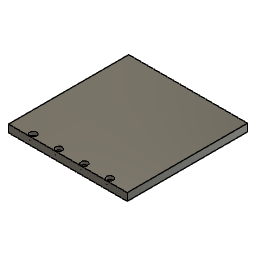
PlaceHeadCover v3 (Autodesk Fusion 360 design; units mm, degrees)
Autodesk Fusion 360 part; units mm, degrees
sketch "Sketch1" plane through (0, 0, 0) normal (0, 1, 0) x (1, 0, 0)
  line L0 (0, 0) -> (79, 0)
  line L1 (79, 0) -> (79, -80)
  line L2 (79, -80) -> (0, -80)
  line L3 (0, -80) -> (0, 0)
  dimension "d1" = 79
  dimension "d2" = 80
  constraint horizontal L0
  constraint vertical L1
  constraint horizontal L2
  constraint vertical L3
  constraint coincident L0.start L3.end
  measures "d1" distance of L0.start L0.end
  measures "d2" distance of L0.start L2.end
extrude "Extrude1" add sketch "Sketch1" along normal blind 5
sketch "Sketch2" plane through (0, 5, 0) normal (0, 1, 0) x (-1, 0, 0)
  line L0 (0, 80) -> (-79, 80)
  line L1 (-79, 80) -> (-79, 0)
  line L2 (-79, 0) -> (0, 0)
  line L3 (0, 0) -> (0, 80)
  point P0 (-14, 77.5)
  dimension "d5" = 14
  dimension "d6" = 2.5
  measures "d5" distance of L3 P0
  measures "d6" distance of L0 P0
hole "Hole1" at (14, 5, 77.5) direction (0, -1, 0) diameter 2 end through all counterbore diameter 4.4 counterbore depth 2.2
pattern_linear "R-Pattern1" count 1 spacing 0 along (0, 0, -1) count 4 spacing 17 along (1, 0, 0) of "Hole1"
